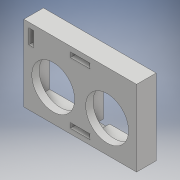
# Autodesk Inventor part: buttons
Saved by Autodesk Inventor 2018 (Build 220112000, 112)
## iProperties
Created: 2018-06-07
Part Number: buttons
Material: Generic
Document SubType Name: Modeling
Designer: bitbots
Density: 1 g/cm^3
Appearance: Default
Author: bitbots
Autodesk Inventor part; units mm, degrees
ref_plane "YZ Plane" through (0, 0, 0) normal (1, 0, 0) x (0, 1, 0)
ref_plane "XZ Plane" through (0, 0, 0) normal (0, 1, 0) x (-1, 0, 0)
ref_plane "XY Plane" through (0, 0, 0) normal (0, 0, 1) x (1, 0, 0)
sketch "Sketch1" plane through (0, 0, 0) normal (0, 1, 0) x (-1, 0, 0)
  line L0 (-23, 13) -> (23, 13)
  line L1 (23, 13) -> (23, -13)
  line L2 (23, -13) -> (-23, -13)
  line L3 (-23, -13) -> (-23, 13)
  line L4 (-23, 13) -> (23, -13) construction
  line L5 (23, 13) -> (-23, -13) construction
  line L6 (0, 0) -> (-11, 0)
  circle A0 centre (-11, 0) radius 8.75
  line L7 (0, 0) -> (11, 0)
  circle A1 centre (11, 0) radius 8.75
  dimension "d0" = 46
  dimension "d1" = 26
  dimension "d2" = 11
  dimension "d3" = 17.5
  dimension "d4" = 11
  dimension "d5" = 17.5
  constraints: 16 end point, 3 horizontal, 2 centre point, 2 coincident, 2 midpoint, 2 parallel, 1 perpendicular
  measures "d0" distance of L1.end L2.end
  measures "d1" distance of L0.end L1.end
  measures "d2" distance of L6.start L6.end
  measures "d3" diameter of A0
  measures "d4" distance of L6.start L7.end
  measures "d5" diameter of A1
extrude "Extrusion1" add sketch "Sketch1" along normal blind 5
sketch "Sketch3" plane through (-23, 0, 13) normal (0, 0, 1) x (1, 0, 0)
  line L0 (46, 0) -> (0, 0) projected
  line L1 (46, 0) -> (46, 5) projected
  line L2 (0, 5) -> (46, 5) projected
  line L3 (0, 0) -> (0, 5) projected
  point P0 (23, 0)
extrude "Extrusion2" add sketch "Sketch3" along normal blind 5
sketch "Sketch2" plane through (0, 5, 0) normal (0, 1, 0) x (1, 0, 0)
  circle A0 centre (-11, 0) radius 8.75 projected
  circle A1 centre (11, 0) radius 8.75 projected
  line L0 (23, 13) -> (23, -18) projected
  line L1 (23, 13) -> (-23, 13) projected
  line L2 (-23, 13) -> (-23, -18) projected
  line L3 (23, 13) -> (-23, 13) projected
  line L4 (0, 13) -> (0, 10)
  line L5 (-4, 9) -> (4, 9)
  line L6 (4, 9) -> (4, 11)
  line L7 (4, 11) -> (-4, 11)
  line L8 (-4, 11) -> (-4, 9)
  line L9 (-4, 9) -> (4, 11) construction
  line L10 (4, 9) -> (-4, 11) construction
  line L11 (23, -18) -> (-23, -18) projected
  line L12 (23, -18) -> (-23, -18) projected
  line L13 (0, -18) -> (0, -15)
  line L14 (-4, -16) -> (4, -16)
  line L15 (4, -16) -> (4, -14)
  line L16 (4, -14) -> (-4, -14)
  line L17 (-4, -14) -> (-4, -16)
  line L18 (-4, -16) -> (4, -14) construction
  line L19 (4, -16) -> (-4, -14) construction
  line L20 (-23, 13) -> (-23, -18) projected
  line L21 (-23, -18) -> (-23, -13)
  line L22 (-23, -13) -> (-20, -13)
  line L23 (-21, -16) -> (-19, -16)
  line L24 (-19, -16) -> (-19, -10)
  line L25 (-19, -10) -> (-21, -10)
  line L26 (-21, -10) -> (-21, -16)
  line L27 (-21, -16) -> (-19, -10) construction
  line L28 (-19, -16) -> (-21, -10) construction
  point P0 (0, 0)
  dimension "d8" = 3
  dimension "d9" = 8
  dimension "d10" = 2
  dimension "d16" = 3
  dimension "d17" = 8
  dimension "d18" = 2
  dimension "d19" = 5
  dimension "d20" = 3
  dimension "d21" = 2
  dimension "d22" = 6
  constraints: 44 end point, 8 midpoint, 6 parallel, 4 perpendicular, 3 horizontal, 2 vertical, 1 point on line
  measures "d8" distance of L4.start L4.end
  measures "d9" distance of L7.end L6.end
  measures "d10" distance of L6.end L5.end
  measures "d16" distance of L13.start L13.end
  measures "d17" distance of L16.end L15.end
  measures "d18" distance of L15.end L14.end
  measures "d19" distance of L2.end L21.end
  measures "d20" distance of L21.end L22.end
  measures "d21" distance of L25.end L24.end
  measures "d22" distance of L24.end L23.end
extrude "Extrusion3" cut sketch "Sketch2" against normal blind 5 contours L7 L6 L5 L8 | L26 L25 L24 L23 | L14 L17 L16 L15
sketch "Sketch4" plane through (0, 5, 0) normal (0, 1, 0) x (1, 0, 0)
  line L0 (4, 11) -> (4, 9) projected
  line L1 (4, 9) -> (-4, 9) projected
  line L2 (-4, 9) -> (-4, 11) projected
  line L3 (-4, 11) -> (4, 11) projected
  line L4 (-19, -10) -> (-19, -16) projected
  line L5 (-19, -16) -> (-21, -16) projected
  line L6 (-21, -16) -> (-21, -10) projected
  line L7 (-21, -10) -> (-19, -10) projected
  line L8 (4, -14) -> (4, -16) projected
  line L9 (4, -16) -> (-4, -16) projected
  line L10 (-4, -16) -> (-4, -14) projected
  line L11 (-4, -14) -> (4, -14) projected
  circle A0 centre (-11, 0) radius 8.75 projected
  circle A1 centre (11, 0) radius 8.75 projected
  line L12 (23, 13) -> (23, -18) projected
  line L13 (23, 13) -> (-23, 13) projected
  line L14 (-23, 13) -> (-23, -18) projected
  line L15 (23, -18) -> (-23, -18) projected
  point P0 (0, 0)
extrude "Extrusion4" add sketch "Sketch4" along normal blind 3
sketch "Sketch5" plane through (0, 8, 0) normal (0, 1, 0) x (1, 0, 0)
  circle A0 centre (11, 0) radius 8.75 projected
  circle A1 centre (-11, 0) radius 8.75 projected
  line L0 (4, -16) -> (-4, -16) projected
  line L1 (-4, -16) -> (-4, -14) projected
  line L2 (-4, -14) -> (4, -14) projected
  line L3 (4, -14) -> (4, -16) projected
  line L4 (4, 9) -> (-4, 9) projected
  line L5 (-4, 9) -> (-4, 11) projected
  line L6 (-4, 11) -> (4, 11) projected
  line L7 (4, 11) -> (4, 9) projected
  line L8 (-19, -16) -> (-21, -16) projected
  line L9 (-21, -16) -> (-21, -10) projected
  line L10 (-21, -10) -> (-19, -10) projected
  line L11 (-19, -10) -> (-19, -16) projected
  line L12 (23, -18) -> (23, 13) projected
  line L13 (23, 13) -> (-23, 13) projected
  line L14 (-23, 13) -> (-23, -18) projected
  line L15 (-23, -18) -> (23, -18) projected
  line L16 (-20.5, -9.5) -> (-1.5, -9.5)
  line L17 (-1.5, -9.5) -> (-1.5, 9.5)
  line L18 (-1.5, 9.5) -> (-20.5, 9.5)
  line L19 (-20.5, 9.5) -> (-20.5, -9.5)
  line L20 (-20.5, -9.5) -> (-1.5, 9.5) construction
  line L21 (-1.5, -9.5) -> (-20.5, 9.5) construction
  line L22 (1.5, -9.5) -> (20.5, -9.5)
  line L23 (20.5, -9.5) -> (20.5, 9.5)
  line L24 (20.5, 9.5) -> (1.5, 9.5)
  line L25 (1.5, 9.5) -> (1.5, -9.5)
  line L26 (1.5, -9.5) -> (20.5, 9.5) construction
  line L27 (20.5, -9.5) -> (1.5, 9.5) construction
  point P0 (0, 0)
  dimension "d27" = 19
  dimension "d28" = 19
  dimension "d29" = 19
  dimension "d30" = 19
  constraints: 24 end point, 4 midpoint, 4 parallel, 2 horizontal, 2 perpendicular
  measures "d27" distance of L18.end L17.end
  measures "d28" distance of L17.end L16.end
  measures "d29" distance of L24.end L23.end
  measures "d30" distance of L23.end L22.end
extrude "Extrusion5" cut sketch "Sketch5" against normal blind 5 contours A0 | A1 | L7 L24 L23 L22 L25 L4 | L4 L25 L24 L7 | L17 L16 L19 L18 L5 L4 | L4 L5 L18 L17
body "Solid1"
